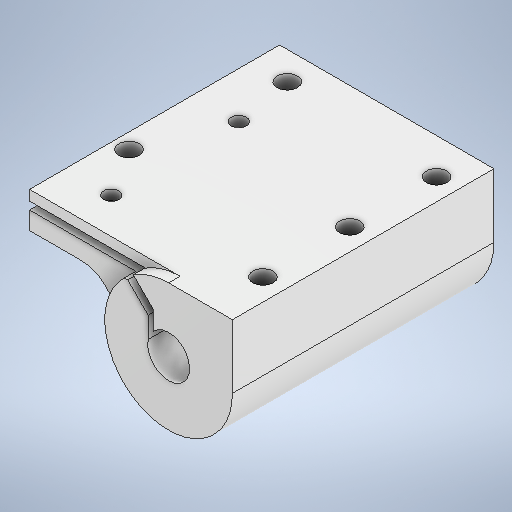
# Autodesk Inventor part: ElevatorShoulderBoltMount
Saved by Autodesk Inventor 2026.2 (Build 302298000, 298)
## iProperties
Created: 2026-03-29
Part Number: ElevatorShoulderBoltMount
Material: ABS Plastic
Document SubType Name: Modeling
Designer: gaoet
Density: 1.06 g/cm^3
Appearance: Smooth - White
Author: gaoet
Autodesk Inventor part; units mm, degrees
ref_plane "YZ Plane" through (0, 0, 0) normal (1, 0, 0) x (0, 1, 0)
ref_plane "XZ Plane" through (0, 0, 0) normal (0, 1, 0) x (-1, 0, 0)
ref_plane "XY Plane" through (0, 0, 0) normal (0, 0, 1) x (1, 0, 0)
sketch "Sketch1" plane through (0, 0, 0) normal (0, 0, 1) x (1, 0, 0)
  circle A0 centre (0, 0) radius 12.5
  circle A1 centre (0, 0) radius 4
  line L0 (12.5, 0) -> (-12.5, 0)
  line L1 (-12.5, 0) -> (-12.5, 12.5)
  line L2 (-12.5, 12.5) -> (12.5, 12.5)
  line L3 (12.5, 12.5) -> (12.5, 0)
  point P0 (0, 12.5)
  dimension "d0" = 25
  dimension "d1" = 8
  constraints: 8 end point, 2 coincident, 2 horizontal, 2 parallel, 2 vertical, 1 centre point, 1 perpendicular, 3 other
  measures "d1" diameter of A1
extrude "Extrusion1" add sketch "Sketch1" along normal blind 38.5 contours L0 A1 A0 | L1 L2 A0 | A0 L0 A1 | A0 L2 L3
sketch "Sketch2" plane through (0, 0, 0) normal (0, 0, -1) x (-1, 0, 0)
  arc A0 (-12.5, 0) -> (12.5, 0) centre (0, 0) ccw projected
  line L0 (12.5, 12.5) -> (12.5, 0) projected
  line L1 (-12.5, 12.5) -> (12.5, 12.5) projected
  line L2 (-12.5, 0) -> (-12.5, 12.5) projected
  circle A1 centre (0, 0) radius 4 projected
  line L3 (5, 2.8868) -> (5, -2.8868)
  line L4 (5, -2.8868) -> (0, -5.7735)
  line L5 (0, -5.7735) -> (-5, -2.8868)
  line L6 (-5, -2.8868) -> (-5, 2.8868)
  line L7 (-5, 2.8868) -> (0, 5.7735)
  line L8 (0, 5.7735) -> (5, 2.8868)
  line L9 (-5.16, -2.879) -> (-5.16, 2.9791)
  line L10 (-5.16, 2.9791) -> (0, 5.9583)
  line L11 (0, 5.9583) -> (5.16, 2.9791)
  line L12 (5.16, 2.9791) -> (5.16, -2.886)
  line L13 (-5.16, -2.879) -> (-5.16, -11.3853)
  line L14 (5.16, -2.886) -> (5.16, -11.3853)
  dimension "d4" = 10
  dimension "d5" = 0.16
  constraints: 24 end point, 3 vertical, 2 point on circle, 1 coincident, 16 other
  measures "d4" distance between parallel lines of L5 L8
  measures "d5" distance between parallel lines of L6 L9
extrude "Extrusion2" add sketch "Sketch2" along normal blind 5.5 contours L2 L1 L0 A0 L14 L12 L11 L10 L9 L13
sketch "Sketch3" plane through (0, 0, -5.5) normal (0, 0, -1) x (-1, 0, 0)
  line L0 (12.5, 12.5) -> (-12.5, 12.5) projected
  line L1 (-12.5, 12.5) -> (-12.5, 0) projected
  arc A0 (-12.5, 0) -> (-5.16, -11.3853) centre (0, 0) ccw projected
  line L2 (-5.16, -11.3853) -> (-5.16, 2.9791) projected
  line L3 (-5.16, 2.9791) -> (0, 5.9583) projected
  line L4 (0, 5.9583) -> (5.16, 2.9791) projected
  line L5 (5.16, 2.9791) -> (5.16, -11.3853) projected
  arc A1 (5.16, -11.3853) -> (12.5, 0) centre (0, 0) ccw projected
  line L6 (12.5, 0) -> (12.5, 12.5) projected
  line L7 (-5.16, 2.9791) -> (-5.16, -11.3853) projected
  arc A2 (-5.16, -11.3853) -> (5.16, -11.3853) centre (0, 0) ccw projected
  line L8 (5.16, -11.3853) -> (5.16, 2.9791) projected
  line L9 (5.16, 2.9791) -> (0, 5.9583) projected
  line L10 (0, 5.9583) -> (-5.16, 2.9791) projected
  circle A3 centre (0, 0) radius 4 projected
extrude "Extrusion3" add sketch "Sketch3" along normal blind 6 contours L6 A1 L5 L4 L3 L2 A0 L1 L0 | A2 L2 L3 L4 L5 | A3
sketch "Sketch4" plane through (0, 0, -11.5) normal (0, 0, -1) x (-1, 0, 0)
  arc A0 (-12.5, 0) -> (12.5, 0) centre (0, 0) ccw projected
  line L0 (12.5, 0) -> (12.5, 12.5) projected
  line L1 (12.5, 12.5) -> (-12.5, 12.5) projected
  line L2 (-12.5, 12.5) -> (-12.5, 0) projected
  line L3 (12.5, 12.5) -> (29.5, 12.5)
  line L4 (29.5, 12.5) -> (29.5, 5.5)
  line L5 (29.5, 5.5) -> (12.5, 5.5)
  line L6 (12.5, 5.5) -> (12.5, 12.5)
  dimension "d10" = 7
  dimension "d11" = 42
  constraints: 8 end point, 2 parallel, 1 horizontal, 1 perpendicular
  measures "d10" distance of L3.end L4.end
  measures "d11" distance of L3.end L1.end
extrude "Extrusion4" add sketch "Sketch4" against normal up to surface (50 mm away) contours L0 L3 L4 L5
fillet "Fillet1" radius 7 1 edges at (-12.5, 5.5, 13.5)
sketch "Sketch5" plane through (0, 0, 38.5) normal (0, 0, 1) x (1, 0, 0)
  arc A0 (-12.463, -0.9615) -> (12.5, 0) centre (0, 0) ccw projected
  line L0 (12.5, 0) -> (12.5, 12.5) projected
  line L1 (12.5, 12.5) -> (-29.5, 12.5) projected
  line L2 (-29.5, 5.5) -> (-29.5, 12.5) projected
  line L3 (-19.4422, 5.5) -> (-29.5, 5.5) projected
  arc A1 (-12.463, -0.9615) -> (-19.4422, 5.5) centre (-19.4422, -1.5) ccw projected
  circle A2 centre (0, 0) radius 4 projected
  line L4 (-4, 0) -> (-4, 9)
  line L5 (-4, 9) -> (-29.5, 9)
  line L6 (-3, 2.6458) -> (-3, 10.5)
  line L7 (-3, 10.5) -> (-29.5, 10.5)
  circle A3 centre (0, 0) radius 4 projected
  dimension "d15" = 1
  dimension "d16" = 1.5
  dimension "d17" = 2
  constraints: 8 end point, 2 perpendicular, 2 point on circle, 2 vertical, 1 midpoint, 1 point on line, 1 tangent
  measures "d15" distance between parallel lines of L4 L6
  measures "d16" distance between parallel lines of L7 L5
  measures "d17" distance between parallel lines of L1 L7
extrude "Extrusion5" cut sketch "Sketch5" against normal up to surface (38.5 mm away) contours L2 L7 L6 A2 L4 L5
sketch "Sketch6" plane through (-29.5, 5.5, -11.5) normal (-1, 0, 0) x (0, 0, 1)
  line L0 (11.5, 5) -> (50, 5) projected
  line L1 (50, 5) -> (50, 7) projected
  line L2 (0, 7) -> (50, 7) projected
  line L3 (0, 0) -> (0, 7) projected
  line L4 (0, 0) -> (50, 0) projected
  line L5 (50, 0) -> (50, 3.5) projected
  line L6 (50, 3.5) -> (11.5, 3.5) projected
  line L7 (11.5, 3.5) -> (11.5, 5) projected
  line L8 (11.5, 5) -> (11, 5)
  line L9 (11, 5) -> (11, -20.7385)
  line L10 (11, -20.7385) -> (11.5, -20.7385)
  line L11 (11.5, -20.7385) -> (11.5, 5)
  point P0 (11.5, -5.5)
  point P1 (11.5, 0)
  point P2 (11, 0)
  dimension "d20" = 0.5
  constraints: 8 end point, 2 parallel, 1 horizontal, 1 perpendicular
  measures "d20" distance between parallel lines of L9 L11
extrude "Extrusion6" cut sketch "Sketch6" against normal up to surface (26.5 mm away) contours L7 L11 L4 L9 L8 | L11 L10 L9 L4
sketch "Sketch7" plane through (-29.5, 5.5, 0) normal (0, -1, 0) x (1, 0, 0)
  line L0 (0, 0) -> (10.0578, 0) projected
  line L1 (10.0578, 38.5) -> (10.0578, 0) projected
  line L2 (10.0578, 38.5) -> (0, 38.5) projected
  line L3 (0, 0) -> (0, 38.5) projected
  circle A0 centre (3, 21) radius 2
  circle A1 centre (3, 21) radius 3
  line L4 (3, 18) -> (0, 18)
  line L5 (3, 24) -> (0, 24)
  point P0 (29.5, 0)
  dimension "d23" = 4
  dimension "d24" = 3
  dimension "d25" = 17.5
  constraints: 4 end point, 3 tangent, 2 centre point, 2 horizontal, 2 point on circle, 2 point on line, 1 coincident
  measures "d23" diameter of A0
  measures "d24" distance from line of L3 A0.centre
  measures "d25" vertical distance of L2.end A0.centre
extrude "Extrusion7" add sketch "Sketch7" against normal up to surface (5 mm away) contours L3 A1 L4 | L3 L5 A1 | A1 | A0
sketch "Sketch8" plane through (-29.5, 5.5, 0) normal (0, -1, 0) x (1, 0, 0)
  circle A0 centre (3, 21) radius 3 projected
  line L0 (3, 24) -> (0, 24) projected
  line L1 (3, 18) -> (0, 18) projected
  circle A1 centre (3, 21) radius 3.5
  line L2 (3, 24.5) -> (-2, 24.5)
  line L3 (3, 17.5) -> (-2, 17.5)
  line L4 (0, 0) -> (0, 38.5) projected
  line L5 (0, 0) -> (10.0578, 0) projected
  line L6 (10.0578, 38.5) -> (10.0578, 0) projected
  line L7 (10.0578, 38.5) -> (0, 38.5) projected
  point P0 (29.5, 0)
  point P1 (0, 17.5)
  point P2 (0, 24.5)
  point P3 (0, 24)
  dimension "d28" = 0.5
  constraints: 4 end point, 2 parallel, 2 tangent, 1 centre point
  measures "d28" radial gap between concentric circles of A0 A1
extrude "Extrusion8" cut sketch "Sketch8" against normal up to surface (3.5 mm away) contours A0 L0 A1 L1 | L0 L4 L2 A1 | A1 L3 L4 L1
sketch "Sketch9" plane through (-29.5, 5.5, 24) normal (0, -1, 0) x (1, 0, 0)
  line L0 (3, 0) -> (0, 0) projected
  line L1 (0, -6) -> (0, 0) projected
  line L2 (0, -6) -> (3, -6) projected
  arc A0 (3, -6) -> (3, 0) centre (3, -3) ccw projected
  line L3 (10.0578, 14.5) -> (10.0578, -24) projected
  line L4 (10.0578, -24.5) -> (0, -24.5) projected
  line L5 (0, -35.5) -> (0, -24.5) projected
  line L6 (10.0578, -35.5) -> (0, -35.5) projected
  line L7 (10.0578, -24.5) -> (10.0578, -35.5) projected
  line L8 (0, 0.5) -> (3, 0.5) projected
  arc A1 (3, -6.5) -> (3, 0.5) centre (3, -3) ccw projected
  line L9 (3, -6.5) -> (0, -6.5) projected
  line L10 (0, -24) -> (0, -6.5) projected
  line L11 (0, -24) -> (10.0578, -24) projected
  line L12 (10.0578, 14.5) -> (0, 14.5) projected
  line L13 (0, 0.5) -> (0, 14.5) projected
  point P0 (29.5, -24)
hole "Hole1" at (-26.5, 5.5, 21) direction (0, 1, 0) diameter 4 depth 7
chamfer "Chamfer1" distance 3.5 angle 45 6 edges at (-28, 9, 24.5) (-23, 9, 21) (-28, 9, 17.5) (-28, 10.5, 24) (-23.5, 10.5, 21) (-28, 10.5, 18)
sketch "Sketch10" plane through (12.5, 12.5, 38.5) normal (0, 1, 0) x (1, 0, 0)
  line L0 (-42, 50) -> (0, 50) projected
  line L1 (-15.5, 0) -> (-15.5, 38.5) projected
  line L2 (-15.5, 38.5) -> (-16.5, 38.5) projected
  line L3 (-16.5, 0) -> (-16.5, 38.5) projected
  line L4 (-15.5, 0) -> (-16.5, 0) projected
  line L5 (0, 0) -> (-42, 0) projected
  line L6 (0, 50) -> (0, 0) projected
  line L7 (-42, 50) -> (0, 50) projected
  line L8 (-42, 50) -> (-42, 0) projected
  line L9 (-8.5, 0) -> (-8.5, 38.5) projected
  point P0 (-12.5, 38.5)
  point P1 (-4.25, 9)
  point P2 (-4.25, 26)
  point P3 (-35, 44.5)
  point P4 (-4.25, 43)
  point P5 (-42, 39)
  dimension "d41" = 17
  dimension "d42" = 50
  dimension "d43" = 17
  dimension "d44" = 9
  dimension "d45" = 11
  dimension "d46" = 5.5
  dimension "d47" = 8.5
  dimension "d48" = 4.25
  constraints: 2 vertical alignment
  measures "d41" distance of point (-4.25, 26) point (-4.25, 9)
  measures "d42" distance of L6.start L5.start
  measures "d43" distance of point (-4.25, 26) point (-4.25, 43)
  measures "d44" distance from line of L5 point (-4.25, 9)
  measures "d45" distance of L0.start point (-42, 39)
  measures "d46" distance from line of L0 point (-35, 44.5)
  measures "d47" distance between parallel lines of L6 L9
  measures "d48" distance from line of L9 point (-4.25, 9)
hole "Hole2" at (8.25, 12.5, 29.5) at (8.25, 12.5, 12.5) at (-22.5, 12.5, -6) at (8.25, 12.5, -4.5) direction (0, -1, 0) diameter 4 depth 15
chamfer "Chamfer2" distance 4 angle 45 3 edges at (-4, 9, 19.25) (-3, 10.5, 19.25) (-3, 10.5, -0.25)
sketch "Sketch13" plane through (12.5, 12.5, 38.5) normal (0, 1, 0) x (1, 0, 0)
  circle A0 centre (-4.25, 43) radius 2 projected
  circle A1 centre (-35, 44.5) radius 2 projected
  circle A2 centre (-4.25, 26) radius 2 projected
  circle A3 centre (-4.25, 9) radius 2 projected
  circle A4 centre (-39, 17.5) radius 2 projected
  line L0 (0, 0) -> (-42, 0) projected
  line L1 (0, 50) -> (0, 0) projected
  line L2 (-42, 50) -> (0, 50) projected
  line L3 (-42, 50) -> (-42, 0) projected
  point P0 (-12.5, 38.5)
  point P1 (-33, 8)
  point P2 (-33, 33)
  dimension "d61" = 8
  dimension "d62" = 25
  dimension "d63" = 9
  constraints: 1 vertical alignment
  measures "d61" distance from line of L0 point (-33, 8)
  measures "d62" distance of point (-33, 8) point (-33, 33)
  measures "d63" distance from line of L3 point (-33, 8)
hole "Hole3" at (-20.5, 12.5, 30.5) at (-20.5, 12.5, 5.5) direction (0, -1, 0) diameter 3 depth 10
fillet "Fillet2" radius 1 1 edges at (5.16, -11.3853, -2.75)
chamfer "Chamfer3" distance 4 angle 45 2 edges at (-18.75, 9, 0) (-18.25, 10.5, -0.5)
sketch "Sketch15" plane through (-5.16, -11.3853, -5.5) normal (1, 0, 0) x (0, 0, -1)
  line L0 (-5, 14.3644) -> (-5, 0) projected
  line L1 (-5, 0) -> (0, 0) projected
  line L2 (0, 14.3644) -> (0, 0) projected
  line L3 (-5, 14.3644) -> (0, 14.3644) projected
  line L4 (-5, 14.3644) -> (0, 0)
  point P0 (-5.5, 11.3853)
  constraints: 2 end point
extrude "Extrusion10" cut sketch "Sketch15" against normal blind 25.4 contours L4 L1 L0
sketch "Sketch16" plane through (0, 0, 0) normal (0, 0, -1) x (-1, 0, 0)
  line L0 (4, 5) -> (16.8441, 5) projected
  line L1 (4, 5) -> (4, 0) projected
  arc A0 (3, 2.6458) -> (4, 0) centre (0, 0) ccw projected
  line L2 (3, 2.6458) -> (3, 4.2262) projected
  line L3 (3, 4.2262) -> (0, 5.9583) projected
  line L4 (0, 5.9583) -> (-5.16, 2.9791) projected
  line L5 (-5.16, 2.9791) -> (-5.16, -9.711) projected
  arc A1 (-6.6957, -10.5555) -> (-5.16, -9.711) centre (-6.16, -9.711) ccw projected
  arc A2 (-6.6957, -10.5555) -> (12.463, -0.9615) centre (0, 0) ccw projected
  arc A3 (16.8441, 5) -> (12.463, -0.9615) centre (19.4422, -1.5) ccw projected
  line L6 (29.5, 5.5) -> (29.5, 9) projected
  line L7 (29.5, 9) -> (20.5, 9) projected
  line L8 (20.5, 9) -> (8, 9) projected
  line L9 (8, 9) -> (4, 5) projected
  line L10 (4, 5) -> (16.8441, 5) projected
  arc A4 (19.4422, 5.5) -> (16.8441, 5) centre (19.4422, -1.5) ccw projected
  line L11 (19.4422, 5.5) -> (29.5, 5.5) projected
  line L12 (29.4021, 5.5) -> (-22.1552, 5.5)
  point P0 (4.5, 5.5)
  constraints: 2 end point, 1 horizontal, 1 point on line
extrude "Extrusion11" cut sketch "Sketch16" against normal blind 0.5 contours L9 L12 A4 L0 | L0 A3 A2 A1 L5 L4 L12 L3 L2 A0 L1 | L12 L4 L3
sketch "Sketch17" plane through (0, 0, 38.5) normal (0, 0, 1) x (1, 0, 0)
  line L0 (-8, 9) -> (-4, 5) projected
  line L1 (-8, 9) -> (-29.5, 9) projected
  line L2 (-29.5, 5.5) -> (-29.5, 9) projected
  line L3 (-19.4422, 5.5) -> (-29.5, 5.5) projected
  arc A0 (-12.463, -0.9615) -> (-19.4422, 5.5) centre (-19.4422, -1.5) ccw projected
  arc A1 (-12.463, -0.9615) -> (12.5, 0) centre (0, 0) ccw projected
  line L4 (12.5, 0) -> (12.5, 12.5) projected
  line L5 (12.5, 12.5) -> (-29.5, 12.5) projected
  line L6 (-29.5, 10.5) -> (-29.5, 12.5) projected
  line L7 (-29.5, 10.5) -> (-7, 10.5) projected
  line L8 (-3, 6.5) -> (-7, 10.5) projected
  line L9 (-3, 6.5) -> (-3, 2.6458) projected
  arc A2 (-4, 0) -> (-3, 2.6458) centre (0, 0) ccw projected
  line L10 (-4, 0) -> (-4, 5) projected
  circle A3 centre (0, 0) radius 12.5
  point P0 (0, 12.5)
  point P1 (-6.9139, 10.4139)
  point P2 (-8.6747, 9)
  constraints: 1 coincident, 3 other
extrude "Extrusion12" add sketch "Sketch17" along normal blind 1.25 contours L0 L10 A2 L9 L8 A3 A1 L1 | L5 L4 A3
sketch "Sketch18" plane through (0, 0, 39.75) normal (0, 0, 1) x (1, 0, 0)
  line L0 (12.5, 0) -> (12.5, 12.5) projected
  line L1 (12.5, 12.5) -> (0, 12.5) projected
  line L2 (-6.9139, 10.4139) -> (-3, 6.5) projected
  line L3 (-3, 6.5) -> (-3, 2.6458) projected
  arc A0 (-4, 0) -> (-3, 2.6458) centre (0, 0) ccw projected
  line L4 (-4, 0) -> (-4, 5) projected
  line L5 (-4, 5) -> (-8, 9) projected
  line L6 (-8, 9) -> (-8.6747, 9) projected
  arc A1 (-8.6747, 9) -> (12.5, 0) centre (0, 0) ccw projected
  circle A2 centre (0, 0) radius 4.1
  arc A3 (0, 12.5) -> (-6.9139, 10.4139) centre (0, 0) ccw projected
  dimension "d81" = 0.1
  constraints: 1 centre point, 1 coincident
  measures "d81" radial gap between concentric circles of A0 A2
extrude "Extrusion13" cut sketch "Sketch18" against normal up to surface (45.25 mm away) contours A2 L3 A0 L4 | L4 A0 L3 A2
sketch "Sketch19" plane through (0, 0, 39.75) normal (0, 0, 1) x (1, 0, 0)
  arc A0 (-4, 0.9) -> (-3, 2.7946) centre (0, 0) ccw projected
  line L0 (-4, 0.9) -> (-4, 5) projected
  line L1 (-4, 5) -> (-8, 9) projected
  line L2 (-8, 9) -> (-8.6747, 9) projected
  arc A1 (-8.6747, 9) -> (12.5, 0) centre (0, 0) ccw projected
  line L3 (12.5, 0) -> (12.5, 12.5) projected
  line L4 (12.5, 12.5) -> (0, 12.5) projected
  line L5 (-6.9139, 10.4139) -> (-3, 6.5) projected
  line L6 (-3, 6.5) -> (-3, 2.7946) projected
  circle A2 centre (0, 0) radius 4.1
  arc A3 (0, 12.5) -> (-6.9139, 10.4139) centre (0, 0) ccw projected
  constraints: 1 coincident, 3 other
extrude "Extrusion14" cut sketch "Sketch19" against normal through all contours A2 A0
sketch "Sketch20" plane through (0, 0, 38.5) normal (0, 0, 1) x (1, 0, 0)
  arc A0 (0, 12.5) -> (-6.9139, 10.4139) centre (0, 0) ccw projected
  line L0 (0, 12.5) -> (-29.5, 12.5) projected
  line L1 (-29.5, 10.5) -> (-29.5, 12.5) projected
  line L2 (-29.5, 10.5) -> (-7, 10.5) projected
  line L3 (-6.9139, 10.4139) -> (-7, 10.5) projected
  arc A1 (-8.6747, 9) -> (-12.463, -0.9615) centre (0, 0) ccw projected
  line L4 (-8.6747, 9) -> (-29.5, 9) projected
  line L5 (-29.5, 5.5) -> (-29.5, 9) projected
  line L6 (-19.4422, 5.5) -> (-29.5, 5.5) projected
  arc A2 (-12.463, -0.9615) -> (-19.4422, 5.5) centre (-19.4422, -1.5) ccw projected
extrude "Extrusion15" cut sketch "Sketch20" against normal blind 1
sketch "Sketch22" plane through (0, 0, 0.5) normal (0, 0, -1) x (-1, 0, 0)
  arc A0 (3, 2.7946) -> (4, 0.9) centre (0, 0) ccw projected
  line L0 (3, 4.2262) -> (3, 2.7946) projected
  line L1 (0, 5.9583) -> (3, 4.2262) projected
  line L2 (-5.16, 2.9791) -> (0, 5.9583) projected
  line L3 (-5.16, -9.711) -> (-5.16, 2.9791) projected
  arc A1 (-6.6957, -10.5555) -> (-5.16, -9.711) centre (-6.16, -9.711) ccw projected
  arc A2 (-6.6957, -10.5555) -> (12.463, -0.9615) centre (0, 0) ccw projected
  arc A3 (19.4422, 5.5) -> (12.463, -0.9615) centre (19.4422, -1.5) ccw projected
  line L4 (4.5, 5.5) -> (19.4422, 5.5) projected
  line L5 (4, 5) -> (4.5, 5.5) projected
  line L6 (4, 0.9) -> (4, 5) projected
  line L7 (19.4422, 5.5) -> (29.5, 5.5) projected
  line L8 (29.5, 5.5) -> (29.5, -12.5)
  line L9 (29.5, -12.5) -> (0, -12.5)
  arc A4 (-6.6957, -10.5555) -> (12.463, -0.9615) centre (0, 0) ccw projected
  arc A5 (-12.5, 0) -> (12.463, -0.9615) centre (0, 0) ccw projected
  line L10 (29.5, 5.5) -> (29.5, 6.9937)
  line L11 (29.5, 6.9937) -> (4, 6.9937)
  line L12 (4, 6.9937) -> (4, 5)
  point P0 (0, -12.5)
  constraints: 10 end point, 3 vertical, 2 horizontal, 1 point on circle, 1 point on line, 1 tangent
extrude "Extrusion16" cut sketch "Sketch22" against normal blind 1
equation "\"d43\" = d41"
equation "\"d46\" = 0.5 * d45"
equation "\"d48\" = 0.5 * d47"
body "Solid1"
